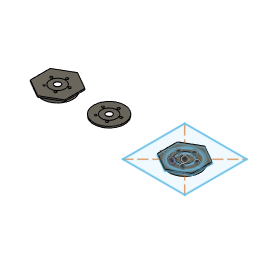
2023_05_26_V_Backup (Autodesk Fusion 360 design; units mm, degrees)
Autodesk Fusion 360 part; units mm, degrees
sketch "Sketch1" plane through (0, 0, 0) normal (0, 0, 1) x (1, 0, 0)
  line L0 (0, 0) -> (13.3, 0) construction
  line L1 (7, 0) -> (-2.725, 0) construction
  line L2 (7, 0) -> (16.725, 0) construction
  line L3 (-2.725, 0) -> (0, 0)
  line L4 (13.3, 0) -> (16.725, 0)
  circle A0 centre (-1.3625, 0) radius 1.3625
  circle A1 centre (15.0125, 0) radius 1.7125
  line L5 (-1.3625, 0) -> (15.0125, 0) construction
  line L6 (15.0125, 0) -> (20.0727, 15.5736) construction
  line L7 (20.0727, 15.5736) -> (6.825, 25.1985) construction
  line L8 (6.825, 25.1985) -> (-6.4227, 15.5736) construction
  line L9 (-6.4227, 15.5736) -> (-1.3625, 0) construction
  circle A2 centre (20.0727, 15.5736) radius 1.7125
  circle A3 centre (6.825, 25.1985) radius 1.7125
  circle A4 centre (-6.4227, 15.5736) radius 1.7125
  circle A5 centre (6.825, 11.2691) radius 4.35
  circle A6 centre (6.825, 11.2691) radius 19.15
  circle A7 centre (6.825, 11.2691) radius 20.5
  circle A8 centre (6.825, 11.2691) radius 22.25
  circle A9 centre (6.825, 11.2691) radius 10.5
  point P0 (6.825, 11.2691)
  dimension "d1" = 13.3
  dimension "d2" = 9.725
  dimension "d3" = 9.725
  dimension "d4" = 8.7
  dimension "d5" = 38.3
  dimension "d6" = 41
  dimension "d7" = 44.5
  dimension "d8" = 21
  constraint coincident L0.start L3.end
  constraint horizontal L0
  constraint coincident L0 L1.start
  constraint parallel L0 L1
  constraint parallel L0 L2
  constraint equal L1 L2
  constraint midpoint L3 A0.centre
  constraint coincident L0.start A0
  constraint midpoint L4 A1.centre
  constraint coincident L0.end A1
  constraint coincident A1.centre L5.end
  constraint coincident A0.centre L5.start
  constraint coincident L6.end L7.start
  constraint coincident L7.end L8.start
  constraint coincident L8.end L9.start
  constraint equal A1 A2
  constraint equal A1 A3
  constraint equal A1 A4
  constraint coincident P0 A5.centre
  constraint concentric A7 A8
  constraint concentric A5 A9
  measures "d1" distance of L0.start L0.end
  measures "d2" distance of L1.start L1.end
  measures "d3" distance of L1.start L2.end
  measures "d4" diameter of A5
  measures "d5" diameter of A6
  measures "d6" diameter of A7
  measures "d7" diameter of A8
  measures "d8" diameter of A9
extrude "Extrude1" add sketch "Sketch1" along normal blind 1.15 contours A9 makes body 1
extrude "Extrude9" add sketch "Sketch1" against normal blind 7.6 contours L3 A0 | L3 A0 | L4 A1 | L4 A1 | A2 | A3 | A4 | A6 | A7 | A8 | A9 bodies 1
extrude "Extrude10" cut sketch "Sketch1" against normal blind 6.5 contours A8 bodies 1
extrude "Extrude11" cut sketch "Sketch1" against normal blind 4.8 contours A7 bodies 1
draft "Draft1" angle 14 neutral plane through (0, 0, 0) pull (0, 0, 1) 1 faces at (-12.2298, 13.1759, -1.6) on bodies 1
extrude "Extrude12" cut sketch "Sketch1" against normal blind 2.16 contours A7 bodies 1
sketch "Sketch2" plane through (0, 0, 0) normal (0, 0, 1) x (1, 0, 0)
  circle A0 centre (6.825, 25.1986) radius 1.35
  circle A1 centre (6.825, 25.1986) radius 2.7
  dimension "d19" = 2.7
  dimension "d20" = 5.4
  constraint concentric A0 A1
  measures "d19" diameter of A0
  measures "d20" diameter of A1
extrude "Extrude6" add sketch "Sketch2" along normal blind 10.76 separate body contours A0 | A1 makes body 2
extrude "Extrude7" cut sketch "Sketch2" along normal blind 7.76 bodies 2
pattern_circular "C-Pattern1" count 5 over 360 about axis through (6.825, 11.2691, 1.15) along (0, 0, -1) of bodies 2 makes body 3 at (19.5298, 16.8096, 5.1733) makes body 4 at (13.9613, -0.847, 2.5867) makes body 5 at (-2.4138, 0.8469, 5.1733) makes body 6 at (-5.942, 16.8351, 5.1733)
move_body "Move3" bodies 6 5 4 3 2 to x (1, 0, 0) y (0, 1, 0) z (0, 0, 1) at (0, 0, 1.3)
extrude "Extrude13" cut sketch "Sketch1" against normal blind 6.5 contours L3 A0 | L3 A0 | L4 A1 | L4 A1 | A2 | A3 | A4 bodies 1
move_body "Move2" bodies 2 to x (1, 0, 0) y (0, 1, 0) z (0, 0, 1) at (0, 0, 1.2)
move_body "Move4" bodies 5 4 6 3 2 to x (1, 0, 0) y (0, 1, 0) z (0, 0, 1) at (0, 0, -7.8)
sketch "Surface Bottom Imac" plane through (0, 0, 0) normal (0, 0, 1) x (1, 0, 0)
  circle A0 centre (6.825, 11.2691) radius 19.15
  circle A1 centre (6.825, 11.2691) radius 10.5
  circle A2 centre (-6.4227, 15.5736) radius 1.7125
  circle A3 centre (-1.3625, 0) radius 1.3625
  circle A4 centre (15.0125, 0) radius 1.7125
  circle A5 centre (20.0727, 15.5736) radius 1.7125
  circle A6 centre (6.825, 25.1985) radius 1.7125
  dimension "d47" = 38.3
  dimension "d48" = 21
  constraint equal A4 A5
  constraint equal A4 A6
  constraint equal A2 A4
  measures "d47" diameter of A0
  measures "d48" diameter of A1
sketch "Sketch4" plane through (0, 0, 0) normal (0, 0, 1) x (1, 0, 0)
sketch "Sketch5" plane through (0, 0, 0) normal (0, 0, 1) x (1, 0, 0)
  circle A0 centre (6.825, 11.2691) radius 19.15
  line L0 (-38.175, -33.7309) -> (51.825, -33.7309)
  line L1 (51.825, -33.7309) -> (51.825, 56.2691)
  line L2 (51.825, 56.2691) -> (-38.175, 56.2691)
  line L3 (-38.175, 56.2691) -> (-38.175, -33.7309)
  line L4 (-38.175, -33.7309) -> (51.825, 56.2691) construction
  line L5 (51.825, -33.7309) -> (-38.175, 56.2691) construction
  circle A1 centre (6.825, 11.2691) radius 10.5
  circle A2 centre (6.825, 11.2691) radius 11
  line L6 (6.825, -17.7601) -> (31.965, -3.2455)
  line L7 (31.965, -3.2455) -> (31.965, 25.7837)
  line L8 (31.965, 25.7837) -> (6.825, 40.2983)
  line L9 (6.825, 40.2983) -> (-18.315, 25.7837)
  line L10 (-18.315, 25.7837) -> (-18.315, -3.2455)
  line L11 (-18.315, -3.2455) -> (6.825, -17.7601)
  point P0 (6.825, 11.2691)
  point P1 (6.825, 11.2691)
  dimension "d49" = 38.3
  dimension "d50" = 90
  dimension "d51" = 90
  dimension "d54" = 21
  dimension "d55" = 0.5
  constraint horizontal L0
  constraint perpendicular L0 L1
  constraint parallel L0 L2
  constraint parallel L1 L3
  constraint coincident L4 P1
  constraint coincident L5 P1
  constraint coincident P0 A0.centre
  constraint coincident P1 P0
  measures "d49" diameter of A0
  measures "d50" distance of L1.end L2.end
  measures "d51" distance of L0.end L1.end
  measures "d54" diameter of A1
extrude "Extrude14" add sketch "Sketch5" sketch "Surface Bottom Imac" along normal blind 2 separate body contours L0 L1 L2 L3 | L6 L7 L8 L9 L10 L11 of sketch 2 makes body 7
extrude "Extrude15" cut sketch "Sketch5" along normal blind 3 contours A2 bodies 1 7
extrude "Extrude16" add sketch "Sketch5" sketch "Sketch1" along normal blind 0.3 separate body contours A2 of sketch 2 contours A9 makes body 8
move_body "Move5" bodies 8 to x (1, 0, 0) y (0, 1, 0) z (0, 0, 1) at (0, 0, 1.7)
combine "Combine2" operation add target body 7 tool bodies 8
extrude "Extrude17" cut sketch "Sketch1" along normal blind 6 contours L3 A0 | L3 A0 | L4 A1 | L4 A1 | A2 | A3 | A4 | A5 | A6 | A7 | A8 | A9 keep common part bodies 7
copy_body "CopyPasteBodies1" bodies 7 makes body 9
move_body "Move6" bodies 9 to x (1, 0, 0) y (0, 1, 0) z (0, 0, 1) at (-110, 0, 0)
extrude "Extrude18" add sketch "Sketch1" against normal blind 6 contours A8 bodies 7
extrude "Extrude19" add sketch "Sketch5" against normal blind 5 contours L6 L7 L8 L9 L10 L11 bodies 7
extrude "Extrude20" add sketch "Sketch5" along normal blind 2 contours A0 | L6 L7 L8 L9 L10 L11 bodies 7
extrude "Extrude21" cut sketch "Sketch1" along normal blind 200 and the other way blind 200 contours L3 A0 | L3 A0 | L4 A1 | L4 A1 | A2 | A3 | A4 bodies 7
extrude "Extrude22" cut 1 faces at (31.0017, 11.2691, -5) along direction (0, 0, 1) blind 5 on bodies 7 bodies 7
copy_body "CopyPasteBodies2" bodies 7 makes body 10
move_body "Move7" bodies 10 to x (1, 0, 0) y (0, 1, 0) z (0, 0, 1) at (-185, 0, 0)
hidden bodies 1
equation "d2 = ( 19.45 / 2 ) * 1 mm"
equation "d23 = 10.76 mm - 3 mm"
equation "d32 = -7.6 mm + 1.1 mm"
equation "d34 = -7.6 mm + 2.8 mm"
equation "d38 = -7.6 mm + 5.44 mm"
named bodies: "Bottom Imac-G4"
